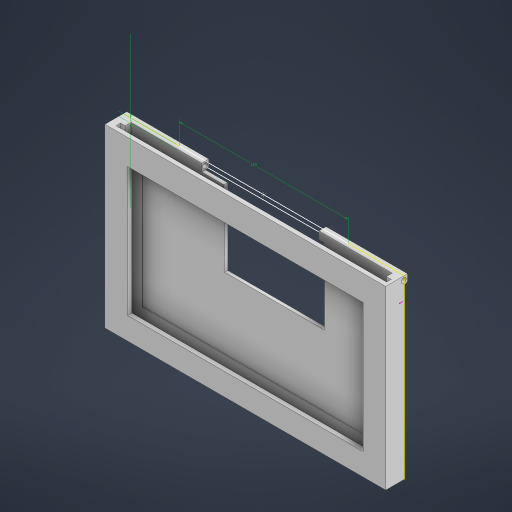
# Autodesk Inventor part: stojan - správná verze
Saved by Autodesk Inventor 2023.3 (Build 273359000, 359)
## iProperties
Created: 2024-01-21
Part Number: stojan - správná verze
Material: Generic
Document SubType Name: Modeling
Designer: matth
Density: 1 g/cm^3
Appearance: Default
Author: matth
Autodesk Inventor part; units mm, degrees
ref_plane "YZ Plane" through (0, 0, 0) normal (1, 0, 0) x (0, 1, 0)
ref_plane "XZ Plane" through (0, 0, 0) normal (0, 1, 0) x (-1, 0, 0)
sketch "Sketch1" plane through (0, 0, 0) normal (0, 0, 1) x (1, 0, 0)
  line L0 (0, 0) -> (183, 0)
  line L1 (183, 0) -> (183, 115)
  line L2 (183, 115) -> (0, 115)
  line L3 (0, 115) -> (0, 0)
  dimension "d0" = 183
  dimension "d1" = 115
  constraints: 8 end point, 2 parallel, 1 horizontal, 1 perpendicular
  measures "d0" distance of L1.end L2.end
  measures "d1" distance of L0.end L1.end
extrude "Extrusion1" add sketch "Sketch1" along normal blind 12
sketch "Sketch2" plane through (0, 115, 0) normal (0, 1, 0) x (1, 0, 0)
  line L0 (0, 0) -> (0, -12) projected
  line L1 (0, -12) -> (183, -12) projected
  line L2 (183, 0) -> (0, 0) projected
  line L3 (7.4669, -2.4521) -> (177.6982, -2.4521)
  line L4 (177.8669, -9.25) -> (7.4669, -9.25)
  line L5 (7.4669, -6.2521) -> (7.4669, -2.4521)
  line L6 (7.4669, -9.2521) -> (7.4669, -9.25)
  line L7 (177.6982, -6.25) -> (177.6982, -2.4521)
  line L8 (7.4669, -9.2521) -> (4.4669, -9.2521)
  line L9 (4.4669, -9.2521) -> (4.4669, -6.2521)
  line L10 (4.4669, -6.2521) -> (7.4669, -6.2521)
  line L11 (177.8669, -9.25) -> (180.8669, -9.25)
  line L12 (180.8669, -9.25) -> (180.8669, -6.25)
  line L13 (180.8669, -6.25) -> (177.6982, -6.25)
  point P0 (0, -6)
  point P1 (0, -6)
  point P2 (0, -6)
  point P3 (0, -6)
  point P4 (91.5, -2.4521)
  point P5 (91.5, 0)
  point P6 (0, -6)
  point P7 (7.3, -9.25)
  dimension "d75" = 170.4
  dimension "d76" = 6.8
  dimension "d122" = 2.75
  dimension "d123" = 6.8
  dimension "d131" = 3
  dimension "d132" = 3
  dimension "d134" = 3
  dimension "d135" = 3
  dimension "d136" = 90
  constraints: 22 end point, 6 midpoint, 4 perpendicular, 3 horizontal, 3 parallel, 2 point on line, 1 vertical alignment
  measures "d75" distance of L4.start L4.end
  measures "d76" distance of L3.end L4.start
  measures "d122" distance between parallel lines of L1 L4
  measures "d123" distance of L3.start L6.start
  measures "d131" distance of L6.start L8.end
  measures "d132" distance of L8.end L9.end
  measures "d134" distance of L4.start L11.end
  measures "d135" distance of L11.end L12.end
  measures "d136" angle of L12 L11
ref_plane "Work Plane1" through (91.5, 0, 0) normal (-1, 0, 0) x (0, 0, 1)
sketch "Sketch6" plane through (91.5, 0, 0) normal (-1, 0, 0) x (0, 0, 1)
  point P0 (0, 115)
  point P1 (0, 101)
sketch "Sketch7" plane through (0, 0, 0) normal (0, 0, -1) x (-1, 0, 0)
  line L0 (-146.5, 112) -> (-36.5, 112)
  line L1 (-36.5, 112) -> (-36.5, 115)
  line L2 (-36.5, 115) -> (-146.5, 115)
  line L3 (-146.5, 115) -> (-146.5, 112)
  line L4 (-183, 115) -> (0, 115) projected
  point P0 (0, 0)
  point P1 (-91.5, 115)
  point P2 (-91.5, 115)
  dimension "d34" = 110
  dimension "d35" = 3
  constraints: 8 end point, 2 midpoint, 2 parallel, 1 horizontal, 1 perpendicular
  measures "d34" distance of L1.end L2.end
  measures "d35" distance of L0.end L1.end
sketch "Sketch14" plane through (0, 0, 12) normal (-1, 0, 0) x (0, 0, 1)
  line L0 (-9, 101) -> (-11, 101) projected
  line L1 (-11, 101) -> (-12, 98.8551)
  line L2 (-12, 0) -> (-12, 115) projected
  line L3 (-9, 101) -> (-6.8161, 101) projected
  line L4 (-9, 101) -> (-11, 101)
  line L5 (-9, 101) -> (-9, 98.8551)
  constraints: 6 end point, 1 horizontal, 1 perpendicular, 2 other
sketch "Sketch15" plane through (183, 0, 12) normal (1, 0, 0) x (0, 0, -1)
  line L0 (11, 101) -> (12, 98.8551) projected
  line L1 (9, 101) -> (11, 101) projected
  line L2 (12, 115) -> (12, 0) projected
  point P0 (12, 0)
  constraints: 1 other
extrude "Extrusion15" cut sketch "Sketch2" against normal blind 110
sketch "Sketch18" plane through (0, 0, 12) normal (0, 0, 1) x (1, 0, 0)
  line L0 (14.75, 98.5) -> (168.25, 98.5)
  line L1 (168.25, 98.5) -> (168.25, 14.5)
  line L2 (168.25, 14.5) -> (14.75, 14.5)
  line L3 (14.75, 14.5) -> (14.75, 98.5)
  line L4 (183, 0) -> (0, 0) projected
  line L5 (0, 115) -> (183, 115) projected
  point P0 (91.5, 98.5)
  point P1 (91.5, 115)
  dimension "d88" = 153.5
  dimension "d89" = 84
  dimension "d90" = 14.5
  constraints: 8 end point, 2 midpoint, 2 parallel, 1 horizontal, 1 perpendicular, 1 vertical alignment
  measures "d88" distance of L1.end L2.end
  measures "d89" distance of L0.end L1.end
  measures "d90" distance between parallel lines of L4 L2
sketch "Sketch19" plane through (0, 115, 0) normal (0, 1, 0) x (1, 0, 0)
  line L0 (183, 0) -> (0, 0) projected
  line L1 (7.4669, -2.4521) -> (177.6982, -2.4521) projected
  line L2 (129.8823, -2.4521) -> (129.8823, 0)
  line L3 (53.4515, -2.4521) -> (53.4515, 0)
  line L4 (129.8823, -2.4521) -> (53.4515, -2.4521)
  line L5 (53.4515, 0) -> (129.8823, 0)
  point P0 (53.4515, 0)
  point P1 (53.4515, -2.4521)
  constraints: 8 end point, 2 collinear, 2 point on line, 1 perpendicular
extrude "Extrusion16" cut sketch "Sketch19" against normal blind 5
sketch "Sketch21" plane through (0, 0, 0) normal (0, 0, -1) x (-1, 0, 0)
  line L0 (-129.8823, 110) -> (-53.4515, 110) projected
  line L1 (0, 115) -> (-183, 115) projected
  line L2 (-53.4515, 110) -> (0, 110)
  line L3 (0, 110) -> (0, 115)
  line L4 (0, 115) -> (-53.4515, 115)
  line L5 (-53.4515, 115) -> (-53.4515, 110)
  line L6 (-183, 0) -> (-183, 115) projected
  line L7 (-183, 115) -> (-129.8898, 115)
  line L8 (-129.8898, 115) -> (-129.8898, 110)
  line L9 (-129.8898, 110) -> (-183, 110)
  line L10 (-183, 110) -> (-183, 115)
  point P0 (0, 0)
  point P1 (-129.8898, 115)
  constraints: 16 end point, 4 parallel, 2 horizontal, 2 perpendicular, 1 point on line
extrude "Extrusion17" add sketch "Sketch21" along normal blind 2.25
sketch "Sketch22" plane through (0, 0, 12) normal (-1, 0, 0) x (0, 0, 1)
  line L0 (-14.25, 115) -> (0, 115) projected
  line L1 (-14.25, 115) -> (-9.25, 115)
  line L2 (-9.25, 115) -> (-9.25, 110)
  line L3 (-12, 110) -> (-14.25, 110) projected
  line L4 (-9.25, 110) -> (-14.25, 110)
  circle A0 centre (-11.75, 112.5) radius 1.6
  point P0 (-12, 0)
  dimension "d95" = 5
  dimension "d96" = 5
  dimension "d97" = 90
  dimension "d98" = 3.2
  constraints: 6 end point, 1 centre point, 1 perpendicular, 1 point on line
  measures "d95" distance of L0.start L1.end
  measures "d96" distance of L1.end L2.end
  measures "d97" angle of L1 L2
  measures "d98" diameter of A0
extrude "Extrusion18" cut sketch "Sketch22" against normal through all
sketch "Sketch23" plane through (0, 0, 0) normal (0, 0, -1) x (-1, 0, 0)
  line L0 (-36.5, 115) -> (-146.5, 115) projected
  line L1 (-183, 110) -> (-129.8898, 110) projected
  line L2 (-133, 110) -> (-68, 110)
  line L3 (-68, 110) -> (-68, 60.5)
  line L4 (-68, 60.5) -> (-133, 60.5)
  line L5 (-133, 60.5) -> (-133, 110)
  line L6 (0, 110) -> (0, 0) projected
  line L7 (-183, 0) -> (-183, 110) projected
  dimension "d101" = 49.5
  dimension "d102" = 68
  dimension "d103" = 50
  constraints: 8 end point, 2 parallel, 1 horizontal, 1 perpendicular, 1 point on line
  measures "d101" distance of L2.end L3.end
  measures "d102" distance between parallel lines of L6 L3
  measures "d103" distance between parallel lines of L7 L5
extrude "Extrusion19" cut sketch "Sketch23" against normal up to surface (9.25 mm away)
sketch "Sketch24" plane through (0, 0, 0) normal (0, 0, -1) x (-1, 0, 0)
  line L0 (-57.7492, 99.1931) -> (-47.7492, 99.1931)
  line L1 (-47.7492, 99.1931) -> (-47.7492, 89.1931)
  line L2 (-47.7492, 89.1931) -> (-57.7492, 89.1931)
  line L3 (-57.7492, 89.1931) -> (-57.7492, 99.1931)
  line L4 (-11.7492, 99.1931) -> (-1.7492, 99.1931)
  line L5 (-1.7492, 99.1931) -> (-1.7492, 89.1931)
  line L6 (-1.7492, 89.1931) -> (-11.7492, 89.1931)
  line L7 (-11.7492, 89.1931) -> (-11.7492, 99.1931)
  line L8 (-57.7492, 21.1931) -> (-47.7492, 21.1931)
  line L9 (-47.7492, 21.1931) -> (-47.7492, 11.1931)
  line L10 (-47.7492, 11.1931) -> (-57.7492, 11.1931)
  line L11 (-57.7492, 11.1931) -> (-57.7492, 21.1931)
  line L12 (-11.7492, 21.1931) -> (-1.7492, 21.1931)
  line L13 (-1.7492, 21.1931) -> (-1.7492, 11.1931)
  line L14 (-1.7492, 11.1931) -> (-11.7492, 11.1931)
  line L15 (-11.7492, 11.1931) -> (-11.7492, 21.1931)
  point P0 (0, 0)
  point P1 (-57.7492, 16.1931)
  point P2 (-57.7492, 94.1931)
  point P3 (-6.7492, 11.1931)
  point P4 (-6.7492, 99.1931)
  dimension "d108" = 10
  dimension "d109" = 10
  dimension "d110" = 10
  dimension "d111" = 10
  dimension "d112" = 10
  dimension "d113" = 10
  dimension "d114" = 10
  dimension "d115" = 10
  dimension "d116" = 56
  dimension "d118" = 88
  dimension "d137" = 88
  constraints: 32 end point, 8 parallel, 4 midpoint, 4 perpendicular, 2 horizontal, 2 point on line, 1 vertical alignment
  measures "d108" distance of L1.end L2.end
  measures "d109" distance of L0.end L1.end
  measures "d110" distance of L5.end L6.end
  measures "d111" distance of L4.end L5.end
  measures "d112" distance of L9.end L10.end
  measures "d113" distance of L8.end L9.end
  measures "d114" distance of L13.end L14.end
  measures "d115" distance of L12.end L13.end
  measures "d116" distance of L4.end L0.start
  measures "d118" distance of L10.end L0.start
  measures "d137" distance of point (-6.749, 11.193) point (-6.749, 99.193)
extrude "Extrusion20" add sketch "Sketch24" along normal blind 5
extrude "Extrusion21" cut sketch "Sketch18" against normal blind 10
chamfer "Chamfer1" distance 1 angle 45 2 edges at (26.7257, 110, -2.25) (156.4449, 110, -2.25)
body "Solid1"
